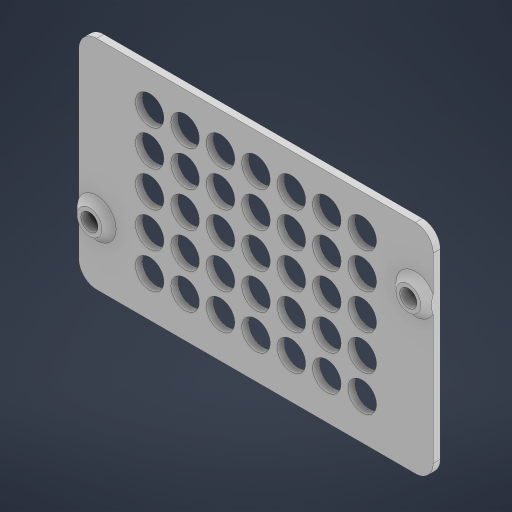
# Autodesk Inventor part: drawer
Saved by Autodesk Inventor 2024 (Build 280153000, 153)
## iProperties
Created: 2024-08-03
Part Number: drawer
Material: Generic
Document SubType Name: Modeling
Designer: micjo
Density: 1 g/cm^3
Appearance: Default
Author: micjo
Autodesk Inventor part; units mm, degrees
ref_plane "YZ Plane" through (0, 0, 0) normal (1, 0, 0) x (0, 1, 0)
ref_plane "XZ Plane" through (0, 0, 0) normal (0, 1, 0) x (-1, 0, 0)
ref_plane "XY Plane" through (0, 0, 0) normal (0, 0, 1) x (1, 0, 0)
sketch "Sketch1" plane through (0, 0, 0) normal (0, 0, 1) x (1, 0, 0)
  line L0 (0, 0) -> (100, 0)
  line L1 (100, 0) -> (100, -61.4)
  line L2 (100, -61.4) -> (0, -61.4)
  line L3 (0, -61.4) -> (0, 0)
  line L4 (0, -61.4) -> (5, -61.4)
  line L5 (5, -61.4) -> (5, -43.9)
  line L6 (5, -43.9) -> (0, -43.9)
  line L7 (0, -43.9) -> (0, -61.4)
  line L8 (5, -43.9) -> (95, -43.9)
  line L9 (95, -43.9) -> (95, -17.5)
  circle A0 centre (5, -43.9) radius 2
  circle A1 centre (95, -17.5) radius 2
  dimension "d0" = 100
  dimension "d1" = 61.4
  dimension "d2" = 5
  dimension "d3" = 17.5
  dimension "d4" = 90
  dimension "d5" = 26.4
  dimension "d6" = 4
  dimension "d7" = 4
  constraints: 20 end point, 5 parallel, 3 perpendicular, 2 centre point, 2 coincident, 2 horizontal
  measures "d0" distance of L1.end L2.end
  measures "d1" distance of L0.end L1.end
  measures "d2" distance of L6.end L5.end
  measures "d3" distance of L5.end L4.end
  measures "d4" distance of L5.end L8.end
  measures "d5" distance of L8.end L9.end
  measures "d6" diameter of A0
  measures "d7" diameter of A1
extrude "Extrusion1" add sketch "Sketch1" along normal blind 2 contours L0 L1 L2 L5 A0 L6 L3 | L6 A0 L5 L2 L3
fillet "Fillet1" radius 5 4 edges at (0, -61.4, 1) (100, -61.4, 1) (0, 0, 1) (100, 0, 1)
sketch "Sketch2" plane through (0, 0, 0) normal (0, 0, -1) x (-1, 0, 0)
  line L0 (0, -60) -> (-10, -60)
  line L1 (-10, -60) -> (-10, 0)
  line L2 (-10, 0) -> (0, 0)
  line L3 (0, 0) -> (0, -60)
  line L4 (-100, -60) -> (-90, -60)
  line L5 (-90, -60) -> (-90, 0)
  line L6 (-90, 0) -> (-100, 0)
  line L7 (-100, 0) -> (-100, -60)
  line L8 (-10, -60) -> (-20, -60)
  line L9 (-20, -60) -> (-20, 0)
  line L10 (-20, 0) -> (-10, 0)
  line L11 (-10, 0) -> (-10, -60)
  line L12 (-20, -60) -> (-30, -60)
  line L13 (-30, -60) -> (-30, 0)
  line L14 (-30, 0) -> (-20, 0)
  line L15 (-20, 0) -> (-20, -60)
  line L16 (-90, -60) -> (-80, -60)
  line L17 (-80, -60) -> (-80, 0)
  line L18 (-80, 0) -> (-90, 0)
  line L19 (-90, 0) -> (-90, -60)
  line L20 (-80, -60) -> (-70, -60)
  line L21 (-70, -60) -> (-70, 0)
  line L22 (-70, 0) -> (-80, 0)
  line L23 (-80, 0) -> (-80, -60)
  line L24 (-70, -60) -> (-60, -60)
  line L25 (-60, -60) -> (-60, 0)
  line L26 (-60, 0) -> (-70, 0)
  line L27 (-70, 0) -> (-70, -60)
  line L28 (-30, -60) -> (-40, -60)
  line L29 (-40, -60) -> (-40, 0)
  line L30 (-40, 0) -> (-30, 0)
  line L31 (-30, 0) -> (-30, -60)
  line L32 (-40, -60) -> (-50, -60)
  line L33 (-50, -60) -> (-50, 0)
  line L34 (-50, 0) -> (-40, 0)
  line L35 (-40, 0) -> (-40, -60)
  line L36 (0, -60) -> (-100, -60)
  line L37 (-100, -60) -> (-100, -50)
  line L38 (-100, -50) -> (0, -50)
  line L39 (0, -50) -> (0, -60)
  line L40 (0, -50) -> (-100, -50)
  line L41 (-100, -50) -> (-100, -40)
  line L42 (-100, -40) -> (0, -40)
  line L43 (0, -40) -> (0, -50)
  line L44 (0, -40) -> (-100, -40)
  line L45 (-100, -40) -> (-100, -30)
  line L46 (-100, -30) -> (0, -30)
  line L47 (0, -30) -> (0, -40)
  line L48 (0, -30) -> (-100, -30)
  line L49 (-100, -30) -> (-100, -20)
  line L50 (-100, -20) -> (0, -20)
  line L51 (0, -20) -> (0, -30)
  line L52 (0, -20) -> (-100, -20)
  line L53 (-100, -20) -> (-100, -10)
  line L54 (-100, -10) -> (0, -10)
  line L55 (0, -10) -> (0, -20)
  circle A0 centre (-20, -50) radius 4
  circle A1 centre (-20, -40) radius 4
  circle A2 centre (-20, -30) radius 4
  circle A3 centre (-20, -20) radius 4
  circle A4 centre (-20, -10) radius 4
  circle A5 centre (-30, -10) radius 4
  circle A6 centre (-30, -20) radius 4
  circle A7 centre (-30, -30) radius 4
  circle A8 centre (-30, -40) radius 4
  circle A9 centre (-30, -50) radius 4
  circle A10 centre (-40, -50) radius 4
  circle A11 centre (-40, -40) radius 4
  circle A12 centre (-40, -30) radius 4
  circle A13 centre (-40, -20) radius 4
  circle A14 centre (-40, -10) radius 4
  circle A15 centre (-50, -10) radius 4
  circle A16 centre (-50, -20) radius 4
  circle A17 centre (-50, -30) radius 4
  circle A18 centre (-50, -40) radius 4
  circle A19 centre (-50, -50) radius 4
  circle A20 centre (-60, -50) radius 4
  circle A21 centre (-60, -40) radius 4
  circle A22 centre (-60, -30) radius 4
  circle A23 centre (-60, -20) radius 4
  circle A24 centre (-60, -10) radius 4
  circle A25 centre (-70, -10) radius 4
  circle A26 centre (-70, -20) radius 4
  circle A27 centre (-70, -30) radius 4
  circle A28 centre (-70, -40) radius 4
  circle A29 centre (-70, -50) radius 4
  circle A30 centre (-80, -50) radius 4
  circle A31 centre (-80, -40) radius 4
  circle A32 centre (-80, -30) radius 4
  circle A33 centre (-80, -20) radius 4
  circle A34 centre (-80, -10) radius 4
  point P0 (0, 0)
  dimension "d11" = 10
  dimension "d12" = 10
  dimension "d13" = 10
  dimension "d14" = 10
  dimension "d15" = 10
  dimension "d16" = 10
  dimension "d17" = 10
  dimension "d18" = 10
  dimension "d19" = 10
  dimension "d20" = 10
  dimension "d21" = 10
  dimension "d22" = 10
  dimension "d23" = 10
  dimension "d24" = 10
  dimension "d25" = 8
  constraints: 102 end point, 37 point on line, 35 centre point, 34 equal radius, 24 parallel, 13 horizontal, 10 perpendicular, 7 midpoint, 4 vertical, 50 other
  measures "d11" distance of L1.end L2.end
  measures "d12" distance of L6.end L5.end
  measures "d13" distance of L9.end L10.end
  measures "d14" distance of L13.end L14.end
  measures "d15" distance of L18.end L17.end
  measures "d16" distance of L22.end L21.end
  measures "d17" distance of L26.end L25.end
  measures "d18" distance of L29.end L30.end
  measures "d19" distance of L33.end L34.end
  measures "d20" distance of L36.end L37.end
  measures "d21" distance of L41.start L41.end
  measures "d22" distance of L45.start L45.end
  measures "d23" distance of L49.start L49.end
  measures "d24" distance of L53.start L53.end
  measures "d25" diameter of A0
extrude "Extrusion2" cut sketch "Sketch2" against normal up to surface (2 mm away) contours A0 L9 L38 | L38 L9 A0 | A0 L38 L9 | A1 L9 L42 | L42 L9 A1 | L38 A0 L9 | A9 L38 L13 | L13 L38 A9 | A2 L9 L46 | L46 L9 A2 | L42 A1 L9 | L9 A1 L42 | L38 L13 A9 | L38 A9 L13 | A10 L38 L29 | L29 L38 A10 | A3 L9 L50 | L50 L9 A3 | L46 A2 L9 | L9 A2 L46 | L38 L29 A10 | L38 A10 L29 | A19 L38 L33 | L33 L38 A19 | A4 L9 L54 | L54 L9 A4 | L50 A3 L9 | L9 A3 L50 | A8 L13 L42 | L42 L13 A8 | A8 L42 L13 | L38 L33 A19 | L38 A19 L33 | A20 L38 L25 | L25 L38 A20 | L54 A4 L9 | L9 A4 L54 | A7 L13 L46 | L46 L13 A7 | L42 A8 L13 | A11 L42 L29 | L29 L42 A11 | L38 L25 A20 | A29 L38 L21 | L21 L38 A29 | L38 A20 L25 | A6 L13 L50 | L50 L13 A6 | L46 A7 L13 | L13 A7 L46 | L42 L29 A11 | L42 A11 L29 | A18 L42 L33 | L33 L42 A18 | A30 L38 L17 | L17 L38 A30 | L38 A29 L21 | L21 A29 L38 | A5 L54 L13 | L13 L54 A5 | A5 L13 L54 | L50 A6 L13 | L13 A6 L50 | L42 L33 A18 | L42 A18 L33 | A21 L42 L25 | L25 L42 A21 | L38 A30 L17 | L17 A30 L38 | L13 A5 L54 | A14 L54 L29 | L29 L54 A14 | A12 L29 L46 | L46 L29 A12 | A12 L46 L29 | L42 L25 A21 | L42 A21 L25 | A28 L42 L21 | L21 L42 A28 | A14 L29 L54 | L29 A14 L54 | A15 L54 L33 | L33 L54 A15 | A13 L29 L50 | L50 L29 A13 | L46 A12 L29 | A17 L46 L33 | L33 L46 A17 | L42 L21 A28 | A31 L17 L42 | L42 L17 A31 | L17 L42 A31 | L42 A28 L21 | A15 L33 L54 | L33 A15 L54 | L50 A13 L29 | L29 A13 L50 | L46 L33 A17 | L46 A17 L33 | A22 L46 L25 | L25 L46 A22 | A32 L17 L46 | L46 L17 A32 | L17 A31 L42 | A24 L25 L54 | L54 L25 A24 | L46 L25 A22 | L46 A22 L25 | A27 L46 L21 | L21 L46 A27 | A33 L17 L50 | L50 L17 A33 | L46 A32 L17 | L17 A32 L46 | A16 L50 L33 | L33 L50 A16 | L54 A24 L25 | L25 A24 L54 | A16 L33 L50 | A16 L50 L33 | L46 L21 A27 | L46 A27 L21 | A34 L17 L54 | L54 L17 A34 | L50 A33 L17 | L17 A33 L50 | A23 L50 L25 | L25 L50 A23 | A23 L50 L25 | L25 L50 A23 | L54 A34 L17 | L17 A34 L54 | A25 L21 L54 | L54 L21 A25 | A26 L50 L21 | L21 L50 A26 | A26 L21 L50 | L54 A25 L21 | L21 A25 L54 | L50 L21 A26
sketch "Sketch3" plane through (0, 0, 2) normal (0, 0, 1) x (1, 0, 0)
  circle A0 centre (5, -43.9) radius 2 projected
  circle A1 centre (5, -43.9) radius 2
  circle A2 centre (95, -17.5) radius 2 projected
  circle A3 centre (95, -17.5) radius 2
  circle A4 centre (5, -43.9) radius 3.5
  circle A5 centre (95, -17.5) radius 3.5
  point P0 (0, 0)
  dimension "d28" = 1.5
  dimension "d29" = 1.5
  constraints: 4 centre point, 2 coincident
  measures "d28" radial gap between concentric circles of A0 A4
  measures "d29" radial gap between concentric circles of A2 A5
extrude "Extrusion3" add sketch "Sketch3" along normal blind 2
sketch "Sketch4" plane through (5, -43.9, 4) normal (0, 0, 1) x (1, 0, 0)
  circle A0 centre (0, 0) radius 2 projected
  circle A1 centre (0, 0) radius 2.4
  circle A2 centre (90, 26.4) radius 2 projected
  circle A3 centre (90, 26.4) radius 2.4
  point P0 (-5, 43.9)
  dimension "d35" = 4.8
  dimension "d36" = 4.8
  constraints: 2 centre point, 2 coincident
  measures "d35" diameter of A1
  measures "d36" diameter of A3
extrude "Extrusion4" cut sketch "Sketch4" against normal up to surface (4 mm away) contours A0 | A1 | A3
chamfer "Chamfer2" distance 2 angle 45 2 edges at (1.5, -43.9, 2) (91.5, -17.5, 2)
body "Solid1"
